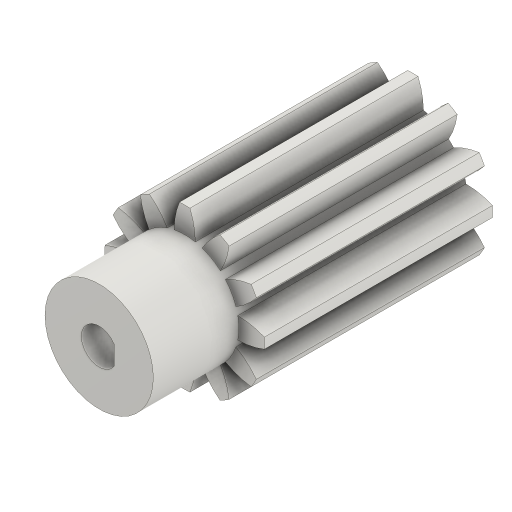
# Autodesk Inventor part: Spur Gear1
Saved by Autodesk Inventor 2024 (Build 280153000, 153)
## iProperties
CustomPartVersion: 1
Created: 2023-07-11
Part Number: Spur Gear1
Material: Steel
Document SubType Name: Modeling
Designer: ferna
Categories: <?xml version="1.0" encoding="UTF-16"?> <MemberInstance><Categories><FamilyTemplate><FamilyTemplateParameter ValueType="xs:double" Id="1" ObjectReferenceKey="da_z" ObjectType="kUserParameterObject"/><FamilyTemplateParameter ValueType="xs:double" Id="2" ObjectReferenceKey="da_b" ObjectType="kUserParameterObject"/><FamilyTemplateParameter ValueType="xs:double" Id="3" ObjectReferenceKey="da_beta" ObjectType="kUserParameterObject"/><FamilyTemplateParameter ValueType="xs:double" Id="4" ObjectReferenceKey="da_da" ObjectType="kUserParameterObject"/><FamilyTemplateParameter ValueType="xs:double" Id="5" ObjectReferenceKey="da_aw" ObjectType="kUserParameterObject"/><FamilyTemplateParameter ValueType="xs:string" Id="6" ObjectReferenceKey="EAIAABAAAACIAQAAAAAAAIAAAAAAAAAA" ObjectType="83910656" SubObjectId="SurfaceGeometry"/></FamilyTemplate><ParamToTemplateMap><ParamToTemplate CategoryParameter="//CategoryParameter[@InternalName='046C89C9-8512-4d59-83FE-43B91F4F132A']" TemplateParameter="1"/><ParamToTemplate CategoryParameter="//CategoryParameter[@InternalName='2552DF32-E462-4b46-AEBF-C6C7768E72AC']" TemplateParameter="2"/><ParamToTemplate CategoryParameter="//CategoryParameter[@InternalName='C9EE641D-15FC-4fae-A226-E94C4372FDD7']" TemplateParameter="3"/><ParamToTemplate><ParamToTemplate CategoryParameter="//CategoryParameter[@InternalName='00B6519A-459B-49c7-AD84-2E56D39A5744']" ConstantValue="0.000000"/></ParamToTemplate><ParamToTemplate><ParamToTemplate CategoryParameter="//CategoryParameter[@InternalName='04B31F0E-C7A6-4894-AA32-9629BEFACF47']" ConstantValue="1.000000"/></ParamToTemplate><ParamToTemplate><ParamToTemplate CategoryParameter="//CategoryParameter[@InternalName='43CBEC2E-7847-49e7-A936-2F7889FCB2D9']" ConstantValue="0.250000"/></ParamToTemplate><ParamToTemplate><ParamToTemplate CategoryParameter="//CategoryParameter[@InternalName='B1EFC894-105D-4ebd-86BF-FA20ED196853']" ConstantValue="0.350000"/></ParamToTemplate><ParamToTemplate><ParamToTemplate CategoryParameter="//CategoryParameter[@InternalName='51175063-3D10-4879-93E8-6246FE8B403D']" ConstantValue="2060000000.000000"/></ParamToTemplate><ParamToTemplate><ParamToTemplate CategoryParameter="//CategoryParameter[@InternalName='A3A52E27-4454-46a9-B0BD-C932399B70AF']" ConstantValue="0.300000"/></ParamToTemplate><ParamToTemplate><ParamToTemplate CategoryParameter="//CategoryParameter[@InternalName='91B76062-C214-41d9-B1B9-14D2AB99603D']" ConstantValue="0.200000"/></ParamToTemplate><ParamToTemplate><ParamToTemplate CategoryParameter="//CategoryParameter[@InternalName='374E806E-8B8A-4dda-A9AA-1039D6500AD2']" ConstantValue="5.000000"/></ParamToTemplate><ParamToTemplate><ParamToTemplate CategoryParameter="//CategoryParameter[@InternalName='2D373A89-B862-43d6-8D0B-0CBF12AB9F6C']" ConstantValue="0.349066"/></ParamToTemplate><ParamToTemplate CategoryParameter="//CategoryParameter[@InternalName='37777632-D6A2-4fac-9D53-DB8ACD95C989']" TemplateParameter="4"/><ParamToTemplate CategoryParameter="//CategoryParameter[@InternalName='FD1017F1-B727-4f7e-9707-0F86F1FF9423']" TemplateParameter="5"/><ParamToTemplate><ParamToTemplate CategoryParameter="//CategoryParameter[@InternalName='9E1B4470-B2D3-4ff1-B813-535BB4CDF51A']" ConstantValue="3520000.000000"/></ParamToTemplate><ParamToTemplate><ParamToTemplate CategoryParameter="//CategoryParameter[@InternalName='F8452263-BFF6-458c-9FB1-07C4B99E95CD']" ConstantValue="11400000.000000"/></ParamToTemplate><ParamToTemplate><ParamToTemplate CategoryParameter="//CategoryParameter[@InternalName='3E3BB259-FD49-497f-8171-6EBC954A3479']" ConstantValue="2.000000"/></ParamToTemplate><ParamToTemplate CategoryParameter="//CategoryParameter[@InternalName='27C3BAF2-7550-4e4b-AE2C-0DB134B7D9B7']" TemplateParameter="6"/></ParamToTemplateMap><Category DisplayName="Gear" InternalName="DC85795E-93AB-48d5-8EEE-5A27447B64BD" Mnemonic="Gear"><CategoryParameter DisplayName="z" InternalName="046C89C9-8512-4d59-83FE-43B91F4F132A" Mnemonic="z"/><CategoryParameter DisplayName="b" InternalName="2552DF32-E462-4b46-AEBF-C6C7768E72AC" Mnemonic="b"/><CategoryParameter DisplayName="||b|" InternalName="C9EE641D-15FC-4fae-A226-E94C4372FDD7" Mnemonic="beta"/><CategoryParameter DisplayName="x" InternalName="00B6519A-459B-49c7-AD84-2E56D39A5744" Mnemonic="x"/><CategoryParameter DisplayName="a*" InternalName="04B31F0E-C7A6-4894-AA32-9629BEFACF47" Mnemonic="a"/><CategoryParameter DisplayName="c*" InternalName="43CBEC2E-7847-49e7-A936-2F7889FCB2D9" Mnemonic="c"/><CategoryParameter DisplayName="r|.f|*" InternalName="B1EFC894-105D-4ebd-86BF-FA20ED196853" Mnemonic="rf"/><CategoryParameter DisplayName="E" InternalName="51175063-3D10-4879-93E8-6246FE8B403D" Mnemonic="E"/><CategoryParameter DisplayName="||m|" InternalName="A3A52E27-4454-46a9-B0BD-C932399B70AF" Mnemonic="mi"/><Category DisplayName="SpurGear" InternalName="26C5A22E-A91E-4dfd-A3B3-23CCAFAE1764" Mnemonic="SpurGear"><CategoryParameter DisplayName="m" InternalName="91B76062-C214-41d9-B1B9-14D2AB99603D" Mnemonic="m"/><CategoryParameter DisplayName="P" InternalName="374E806E-8B8A-4dda-A9AA-1039D6500AD2" Mnemonic="PP"/><CategoryParameter DisplayName="||a|" InternalName="2D373A89-B862-43d6-8D0B-0CBF12AB9F6C" Mnemonic="alpha"/><CategoryParameter DisplayName="d|.a|" InternalName="37777632-D6A2-4fac-9D53-DB8ACD95C989" Mnemonic="da"/><CategoryParameter DisplayName="a|.w|" InternalName="FD1017F1-B727-4f7e-9707-0F86F1FF9423" Mnemonic="aw"/><CategoryParameter DisplayName="||s||.Flim|" InternalName="9E1B4470-B2D3-4ff1-B813-535BB4CDF51A" Mnemonic="sFlim"/><CategoryParameter DisplayName="||s||.Hlim|" InternalName="F8452263-BFF6-458c-9FB1-07C4B99E95CD" Mnemonic="sHlim"/><CategoryParameter DisplayName="type" InternalName="3E3BB259-FD49-497f-8171-6EBC954A3479" Mnemonic="type"/><CategoryParameter DisplayName="PitchDiameter" InternalName="27C3BAF2-7550-4e4b-AE2C-0DB134B7D9B7" Mnemonic="IDS_PITCHDIAM"/></Category></Category></Categories></MemberInstance>
Density: 1 g/cm^3
Appearance: Steel
Author: ferna
Autodesk Inventor part; units mm, degrees
sketch "Sketch1" plane through (0, 0, 0) normal (0, 0, 1) x (1, 0, 0)
  circle A0 centre (0, 0) radius 14
  dimension "d0" = 28
  constraints: 1 centre point
  measures "d0" diameter of A0
extrude "Extrusion1" add sketch "Sketch1" along normal blind 20
ref_plane "Work Plane2" through (0, 0, 10) normal (0, 0, 1) x (1, 0, 0)
sketch "Sketch2" plane through (0, 0, 0) normal (0, 0, -1) x (-1, 0, 0)
  circle A0 centre (0, 0) radius 14 projected
  circle A1 centre (0, 0) radius 12
  dimension "d3" = 24
  constraints: 1 centre point, 1 coincident
  measures "d3" diameter of A1
surface extrude "Pitch Diameter" sketch "Sketch2" against normal through all shown no curves A1
ref_plane "Work Plane8" through (0, 0, 0) normal (0.9659258, 0.258819, 0) x (0, 0, 1)
ref_plane "Work Plane9" through (0, 0, 0) normal (1, 0, 0) x (0, 1, 0)
spur gear teeth "Spur Gear" teeth 12 pitch diameter 24 tip diameter 28 root diameter 19 face width 20 start plane through (0, 0, 0) normal (0, 0, -1) x (-1, 0, 0)
sketch "Sketch3" plane through (0, 0, 20) normal (0, 0, 1) x (1, 0, 0)
  arc A0 (-7.778, 11.6406) -> (-6.2638, 7.1425) centre (4.4642, 13.2578) ccw projected
  arc A1 (-6.2638, 7.1425) -> (-7.1425, 6.2638) centre (0, 0) ccw projected
  arc A2 (-7.1425, 6.2638) -> (-11.6406, 7.778) centre (-13.2578, -4.4642) ccw projected
  arc A3 (-11.6406, 7.778) -> (-12.5562, 6.192) centre (0, 0) ccw projected
  arc A4 (-12.5562, 6.192) -> (-8.9958, 3.0537) centre (-2.7628, 13.7136) ccw projected
  arc A5 (-8.9958, 3.0537) -> (-9.3175, 1.8534) centre (0, 0) ccw projected
  arc A6 (-9.3175, 1.8534) -> (-13.97, 0.9156) centre (-9.2495, -10.495) ccw projected
  arc A7 (-13.97, 0.9156) -> (-13.97, -0.9156) centre (0, 0) ccw projected
  arc A8 (-13.97, -0.9156) -> (-9.3175, -1.8534) centre (-9.2495, 10.495) ccw projected
  arc A9 (-9.3175, -1.8534) -> (-8.9958, -3.0537) centre (0, 0) ccw projected
  arc A10 (-8.9958, -3.0537) -> (-12.5562, -6.192) centre (-2.7628, -13.7136) ccw projected
  arc A11 (-12.5562, -6.192) -> (-11.6406, -7.778) centre (0, 0) ccw projected
  arc A12 (-11.6406, -7.778) -> (-7.1425, -6.2638) centre (-13.2578, 4.4642) ccw projected
  arc A13 (-7.1425, -6.2638) -> (-6.2638, -7.1425) centre (0, 0) ccw projected
  arc A14 (-6.2638, -7.1425) -> (-7.778, -11.6406) centre (4.4642, -13.2578) ccw projected
  arc A15 (-7.778, -11.6406) -> (-6.192, -12.5562) centre (0, 0) ccw projected
  arc A16 (-6.192, -12.5562) -> (-3.0537, -8.9958) centre (-13.7136, -2.7628) ccw projected
  arc A17 (-3.0537, -8.9958) -> (-1.8534, -9.3175) centre (0, 0) ccw projected
  arc A18 (-1.8534, -9.3175) -> (-0.9156, -13.97) centre (10.495, -9.2495) ccw projected
  arc A19 (-0.9156, -13.97) -> (0.9156, -13.97) centre (0, 0) ccw projected
  arc A20 (0.9156, -13.97) -> (1.8534, -9.3175) centre (-10.495, -9.2495) ccw projected
  arc A21 (1.8534, -9.3175) -> (3.0537, -8.9958) centre (0, 0) ccw projected
  arc A22 (3.0537, -8.9958) -> (6.192, -12.5562) centre (13.7136, -2.7628) ccw projected
  arc A23 (6.192, -12.5562) -> (7.778, -11.6406) centre (0, 0) ccw projected
  arc A24 (7.778, -11.6406) -> (6.2638, -7.1425) centre (-4.4642, -13.2578) ccw projected
  arc A25 (6.2638, -7.1425) -> (7.1425, -6.2638) centre (0, 0) ccw projected
  arc A26 (7.1425, -6.2638) -> (11.6406, -7.778) centre (13.2578, 4.4642) ccw projected
  arc A27 (11.6406, -7.778) -> (12.5562, -6.192) centre (0, 0) ccw projected
  arc A28 (12.5562, -6.192) -> (8.9958, -3.0537) centre (2.7628, -13.7136) ccw projected
  arc A29 (8.9958, -3.0537) -> (9.3175, -1.8534) centre (0, 0) ccw projected
  arc A30 (9.3175, -1.8534) -> (13.97, -0.9156) centre (9.2495, 10.495) ccw projected
  arc A31 (13.97, -0.9156) -> (13.97, 0.9156) centre (0, 0) ccw projected
  arc A32 (13.97, 0.9156) -> (9.3175, 1.8534) centre (9.2495, -10.495) ccw projected
  arc A33 (9.3175, 1.8534) -> (8.9958, 3.0537) centre (0, 0) ccw projected
  arc A34 (8.9958, 3.0537) -> (12.5562, 6.192) centre (2.7628, 13.7136) ccw projected
  arc A35 (12.5562, 6.192) -> (11.6406, 7.778) centre (0, 0) ccw projected
  arc A36 (11.6406, 7.778) -> (7.1425, 6.2638) centre (13.2578, -4.4642) ccw projected
  arc A37 (7.1425, 6.2638) -> (6.2638, 7.1425) centre (0, 0) ccw projected
  arc A38 (6.2638, 7.1425) -> (7.778, 11.6406) centre (-4.4642, 13.2578) ccw projected
  arc A39 (7.778, 11.6406) -> (6.192, 12.5562) centre (0, 0) ccw projected
  arc A40 (6.192, 12.5562) -> (3.0537, 8.9958) centre (13.7136, 2.7628) ccw projected
  arc A41 (3.0537, 8.9958) -> (1.8534, 9.3175) centre (0, 0) ccw projected
  arc A42 (1.8534, 9.3175) -> (0.9156, 13.97) centre (-10.495, 9.2495) ccw projected
  arc A43 (0.9156, 13.97) -> (-0.9156, 13.97) centre (0, 0) ccw projected
  arc A44 (-0.9156, 13.97) -> (-1.8534, 9.3175) centre (10.495, 9.2495) ccw projected
  arc A45 (-1.8534, 9.3175) -> (-3.0537, 8.9958) centre (0, 0) ccw projected
  arc A46 (-3.0537, 8.9958) -> (-6.192, 12.5562) centre (-13.7136, 2.7628) ccw projected
  arc A47 (-6.192, 12.5562) -> (-7.778, 11.6406) centre (0, 0) ccw projected
extrude "Extrusion2" add sketch "Sketch3" along normal blind 20
sketch "Sketch4" plane through (0, 0, 40) normal (0, 0, 1) x (1, 0, 0)
  circle A0 centre (0, 0) radius 10
  arc A1 (2.65, 1.6562) -> (2.65, -1.6562) centre (0, 0) ccw
  line L0 (2.65, 1.6562) -> (2.65, -1.6562)
  circle A2 centre (0, 0) radius 9.5
  point P0 (0, 0)
  point P1 (0, 0)
  constraints: 3 centre point, 2 end point, 2 point on circle, 1 coincident
extrude "Extrusion3" add sketch "Sketch4" along normal blind 15 contours A2
equation "\"d0\" = da_da"
equation "\"d1\" = da_b"
equation "\"d3\" = da_d"
equation "\"da_da\" = 28"
equation "\"da_b\" = 20"
equation "\"da_d\" = 24"
body "Solid1"
body "Srf1"
